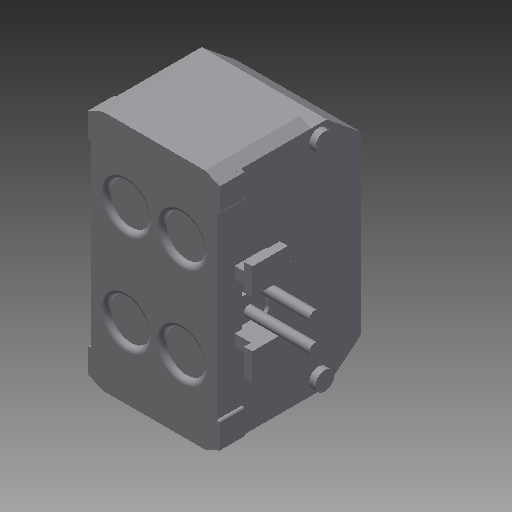
# Autodesk Inventor part: 259434_part2
Saved by Autodesk Inventor 2019.3 (Build 233278000, 278)
## iProperties
Category: PARTsolutions
Company: MOELLER
Created: 2018-11-06
Part Number: 259434_part2
Material: Generic
Catalog Web Link: www.cadenas.de
Description: NZM1-XU_p2-NZM1-XU_p2
Vendor: MOELLER
Document SubType Name: Modeling
Designer: psadmin
Manufacturer: MOELLER
Mass: 17.1132 g
Surface Area: 44.1464 cm^2
Volume: 17.1132 cm^3
Density: 1 g/cm^3
Appearance: PSOLRGB-192-192-192
PSOL_IDENT_0: {$CADENAS_DATA\23d-libs\moeller\circuit_breaker\parts\nzm1_xu_p2.prj},168 {VTYP=3D},{NB=259434_part2
PSOL_IDENT_1: },{LINA=259434_part2},{NN=NZM1-XU_p2},{DATE=05.10.2018 14:14:17},{GEOMDATE=14.05.2018 10:43:06},{VER
PSOL_IDENT_2: SION=},{LINEID=10},{WBVAR=},{WBNUMERIC=}  {NB=259434_part2},{LINA=259434_part2},{KT=DUMMY},{BMENB=25
PSOL_IDENT_3: 9434},{EPLAN=}
NN: NZM1-XU_p2
NT: NZM1-XU_p2
NB: 259434_part2
NBSYN: $BMENB._part2
LINA: 259434_part2
BMENB: 259434
SUPPLIER: MOELLER
ARTICLENO: 259434_part2
BOMINFO: 259434_part2
CREATOR: CADENAS GmbH
Title: 259434_part2
Author: Cadenas PARTsolutions
Comments: NZM1-XU_p2
Autodesk Inventor part; units mm, degrees
sketch "Sketch_1" plane through (0, 0, 0) normal (1, 0, 0) x (0, 1, 0)
  line L0 (-18.5, 0) -> (-18.5, -17.6)
  line L1 (-18.5, -17.6) -> (-14, -23.1)
  line L2 (-14, -23.1) -> (14, -23.1)
  line L3 (14, -23.1) -> (18.5, -17.6)
  line L4 (18.5, -17.6) -> (18.5, 0)
  line L5 (18.5, 0) -> (-18.5, 0)
  constraints: 12 end point
extrude "Extrusion1" add sketch "Sketch_1" along normal blind 20
sketch "Sketch_2" plane through (0, 0, 0) normal (0, 0, 1) x (1, 0, 0)
  line L0 (0, 18.5) -> (20, 18.5)
  line L1 (20, 18.5) -> (18.15, 19.3)
  line L2 (18.15, 19.3) -> (1.85, 19.3)
  line L3 (1.85, 19.3) -> (0, 18.5)
  constraints: 8 end point
extrude "Extrusion2" add sketch "Sketch_2" against normal blind 15.1
sketch "Sketch_3" plane through (0, 0, 0) normal (0, 0, 1) x (1, 0, 0)
  line L0 (0, -18.5) -> (1.85, -19.3)
  line L1 (1.85, -19.3) -> (18.15, -19.3)
  line L2 (18.15, -19.3) -> (20, -18.5)
  line L3 (20, -18.5) -> (0, -18.5)
  constraints: 8 end point
extrude "Extrusion3" add sketch "Sketch_3" against normal blind 15.1
sketch "Sketch_4" plane through (0, 0, 0) normal (0, 0, 1) x (1, 0, 0)
  line L0 (-0.5, 18.272) -> (-0.5, 14.3)
  line L1 (-0.5, 14.3) -> (0.5, 14.3)
  line L2 (0.5, 14.3) -> (0.5, 18.7044)
  line L3 (0.5, 18.7044) -> (-0.5, 18.272)
  constraints: 8 end point
extrude "Extrusion4" add sketch "Sketch_4" against normal blind 4
sketch "Sketch_5" plane through (0, 0, 0) normal (0, 0, 1) x (1, 0, 0)
  line L0 (19.5, 18.7044) -> (19.5, 14.3)
  line L1 (19.5, 14.3) -> (20.1, 14.3)
  arc A0 (20.1, 14.3) -> (20.5, 14.7) centre (20.1, 14.7) ccw
  line L2 (20.5, 14.7) -> (20.5, 18.272)
  line L3 (20.5, 18.272) -> (19.5, 18.7044)
  constraints: 8 end point, 2 point on circle, 1 centre point
extrude "Extrusion5" add sketch "Sketch_5" against normal blind 4
sketch "Sketch_6" plane through (0, 0, 0) normal (0, 0, 1) x (1, 0, 0)
  line L0 (-0.5, -18.272) -> (0.5, -18.7044)
  line L1 (0.5, -18.7044) -> (0.5, -14.3)
  line L2 (0.5, -14.3) -> (-0.5, -14.3)
  line L3 (-0.5, -14.3) -> (-0.5, -18.272)
  constraints: 8 end point
extrude "Extrusion6" add sketch "Sketch_6" against normal blind 4
sketch "Sketch_7" plane through (0, 0, 0) normal (0, 0, 1) x (1, 0, 0)
  line L0 (19.5, -18.7044) -> (20.5, -18.272)
  line L1 (20.5, -18.272) -> (20.5, -14.7)
  arc A0 (20.5, -14.7) -> (20.1, -14.3) centre (20.1, -14.7) ccw
  line L2 (20.1, -14.3) -> (19.5, -14.3)
  line L3 (19.5, -14.3) -> (19.5, -18.7044)
  constraints: 8 end point, 2 point on circle, 1 centre point
extrude "Extrusion7" add sketch "Sketch_7" against normal blind 4
sketch "Sketch_8" plane through (20, 0, 0) normal (1, 0, 0) x (0, 0, -1)
  circle A0 centre (16.3, 16.5) radius 1.5
  constraints: 1 centre point
extrude "Extrusion8" add sketch "Sketch_8" along normal mid plane 2
sketch "Sketch_9" plane through (20, 0, 0) normal (1, 0, 0) x (0, 0, -1)
  circle A0 centre (16.3, -16.5) radius 1.5
  constraints: 1 centre point
extrude "Extrusion9" add sketch "Sketch_9" along normal mid plane 2
sketch "Sketch_10" plane through (5.55, 0, 0) normal (1, 0, 0) x (0, 0, -1)
  line L0 (0.8, 8) -> (-1.2, 8)
  line L1 (-1.2, 8) -> (-1.2, 12.05)
  line L2 (-1.2, 12.05) -> (0, 12.05)
  arc A0 (0, 12.05) -> (0.8, 11.25) centre (0.8, 12.05) ccw
  line L3 (0.8, 11.25) -> (0.8, 8)
  line L4 (0.8, 8) -> (-1.2, 8)
  constraints: 10 end point, 2 point on circle, 1 centre point
revolve "Revolution1" cut sketch "Sketch_10" angle 360 about axis through (5.55, 8, -0.8) along (0, 0, -1)
sketch "Sketch_11" plane through (14.45, 0, 0) normal (1, 0, 0) x (0, 0, -1)
  line L0 (0.8, 8) -> (-1.2, 8)
  line L1 (-1.2, 8) -> (-1.2, 12.05)
  line L2 (-1.2, 12.05) -> (0, 12.05)
  arc A0 (0, 12.05) -> (0.8, 11.25) centre (0.8, 12.05) ccw
  line L3 (0.8, 11.25) -> (0.8, 8)
  line L4 (0.8, 8) -> (-1.2, 8)
  constraints: 10 end point, 2 point on circle, 1 centre point
revolve "Revolution2" cut sketch "Sketch_11" angle 360 about axis through (14.45, 8, -0.8) along (0, 0, -1)
sketch "Sketch_12" plane through (5.55, 0, 0) normal (1, 0, 0) x (0, 0, -1)
  line L0 (0.8, -8) -> (-1.2, -8)
  line L1 (-1.2, -8) -> (-1.2, -3.95)
  line L2 (-1.2, -3.95) -> (0, -3.95)
  arc A0 (0, -3.95) -> (0.8, -4.75) centre (0.8, -3.95) ccw
  line L3 (0.8, -4.75) -> (0.8, -8)
  line L4 (0.8, -8) -> (-1.2, -8)
  constraints: 10 end point, 2 point on circle, 1 centre point
revolve "Revolution3" cut sketch "Sketch_12" angle 360 about axis through (5.55, -8, -0.8) along (0, 0, -1)
sketch "Sketch_13" plane through (14.45, 0, 0) normal (1, 0, 0) x (0, 0, -1)
  line L0 (0.8, -8) -> (-1.2, -8)
  line L1 (-1.2, -8) -> (-1.2, -3.95)
  line L2 (-1.2, -3.95) -> (0, -3.95)
  arc A0 (0, -3.95) -> (0.8, -4.75) centre (0.8, -3.95) ccw
  line L3 (0.8, -4.75) -> (0.8, -8)
  line L4 (0.8, -8) -> (-1.2, -8)
  constraints: 10 end point, 2 point on circle, 1 centre point
revolve "Revolution4" cut sketch "Sketch_13" angle 360 about axis through (14.45, -8, -0.8) along (0, 0, -1)
sketch "Sketch_14" plane through (20, 0, 0) normal (1, 0, 0) x (0, 0, -1)
  line L0 (2.9, 5.6) -> (2.9, 3.75)
  line L1 (2.9, 3.75) -> (7.8, 3.75)
  arc A0 (7.8, 3.75) -> (8.3, 4.25) centre (7.8, 4.25) ccw
  line L2 (8.3, 4.25) -> (8.3, 5.1)
  arc A1 (8.3, 5.1) -> (7.8, 5.6) centre (7.8, 5.1) ccw
  line L3 (7.8, 5.6) -> (2.9, 5.6)
  constraints: 8 end point, 4 point on circle, 2 centre point
extrude "Extrusion10" add sketch "Sketch_14" along normal mid plane 7.8
sketch "Sketch_15" plane through (20, 0, 0) normal (1, 0, 0) x (0, 0, -1)
  line L0 (2.9, -3.75) -> (2.9, -5.6)
  line L1 (2.9, -5.6) -> (7.8, -5.6)
  arc A0 (7.8, -5.6) -> (8.3, -5.1) centre (7.8, -5.1) ccw
  line L2 (8.3, -5.1) -> (8.3, -4.25)
  arc A1 (8.3, -4.25) -> (7.8, -3.75) centre (7.8, -4.25) ccw
  line L3 (7.8, -3.75) -> (2.9, -3.75)
  constraints: 8 end point, 4 point on circle, 2 centre point
extrude "Extrusion11" add sketch "Sketch_15" along normal mid plane 7.8
sketch "Sketch_16" plane through (23.9, 0, 0) normal (1, 0, 0) x (0, 0, -1)
  line L0 (1.8, 3.75) -> (8.0083, 3.75)
  line L1 (8.0083, 3.75) -> (7.5053, 8)
  line L2 (7.5053, 8) -> (1.8, 8)
  line L3 (1.8, 8) -> (1.8, 3.75)
  constraints: 8 end point
extrude "Extrusion12" add sketch "Sketch_16" against normal blind 1.3
sketch "Sketch_17" plane through (23.9, 0, 0) normal (1, 0, 0) x (0, 0, -1)
  line L0 (1.8, -3.75) -> (1.8, -8)
  line L1 (1.8, -8) -> (7.5053, -8)
  line L2 (7.5053, -8) -> (8.0083, -3.75)
  line L3 (8.0083, -3.75) -> (1.8, -3.75)
  constraints: 8 end point
extrude "Extrusion13" add sketch "Sketch_17" against normal blind 1.3
sketch "Sketch_19" plane through (20, 0, 0) normal (1, 0, 0) x (0, 0, -1)
  line L0 (4, 3.75) -> (4, 0.75)
  line L1 (4, 0.75) -> (7.4, 0.75)
  arc A0 (7.4, 0.75) -> (8.4, 1.75) centre (7.4, 1.75) ccw
  line L2 (8.4, 1.75) -> (8.4, 2.75)
  arc A1 (8.4, 2.75) -> (7.4, 3.75) centre (7.4, 2.75) ccw
  line L3 (7.4, 3.75) -> (4, 3.75)
  constraints: 8 end point, 4 point on circle, 2 centre point
extrude "Extrusion14" cut sketch "Sketch_19" along normal mid plane 1.1
sketch "Sketch_20" plane through (20, 0, 0) normal (1, 0, 0) x (0, 0, -1)
  line L0 (4, -0.75) -> (4, -3.75)
  line L1 (4, -3.75) -> (7.4, -3.75)
  arc A0 (7.4, -3.75) -> (8.4, -2.75) centre (7.4, -2.75) ccw
  line L2 (8.4, -2.75) -> (8.4, -1.75)
  arc A1 (8.4, -1.75) -> (7.4, -0.75) centre (7.4, -1.75) ccw
  line L3 (7.4, -0.75) -> (4, -0.75)
  constraints: 8 end point, 4 point on circle, 2 centre point
extrude "Extrusion15" cut sketch "Sketch_20" along normal mid plane 1.1
sketch "Sketch_21" plane through (20, 0, 0) normal (1, 0, 0) x (0, 0, -1)
  circle A0 centre (5.65, 2.25) radius 0.8
  constraints: 1 centre point
extrude "Extrusion16" add sketch "Sketch_21" along normal mid plane 20
sketch "Sketch_22" plane through (20, 0, 0) normal (1, 0, 0) x (0, 0, -1)
  circle A0 centre (5.65, -2.25) radius 0.8
  constraints: 1 centre point
extrude "Extrusion17" add sketch "Sketch_22" along normal mid plane 20
ref_plane "2p1_XY" through (0, 0, 0) normal (0, 0, -1) x (1, 0, 0)
ref_plane "2p1_YZ" through (0, 0, 0) normal (1, 0, 0) x (0, -1, 0)
ref_plane "2p1_ZX" through (0, 0, 0) normal (0, -1, 0) x (0, 0, -1)
body "Solid1"
